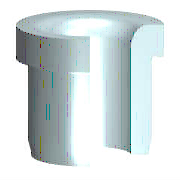
# Autodesk Inventor part: DIN 172 - A 3 x 12
Saved by Autodesk Inventor 2023.3 (Build 273359000, 359)
## iProperties
Created: 2022-02-04
Part Number: DIN 172 - A 3 x 12
Material: Stahl, weich
Description: Bohrbuchse
Document SubType Name: Modeling
Standard: DIN 172
Designer: nicob
Standards Organization: DIN
Language: de-DE
Size Designation: A 3 x 12
Categories: <MemberInstance><Categories><Category DisplayName="Sonstige Bauteile" InternalName="5aa15e00-363f-49f2-933f-16f664388e3f" Mnemonic="OTHER"><Category DisplayName="Bohrbuchsen" InternalName="dee9b2ed-98ff-44bf-b329-c7a8019090da" Mnemonic="BUSH"><CategoryParameter DisplayName="Max. Nenndurchmesser" InternalName="b1ee04ef-1694-415b-b3bc-4245da0f3d9b" Mnemonic="nomdiamax"/><CategoryParameter DisplayName="Nenndurchmesser" InternalName="b4c3aa1f-6c9b-46e9-b968-1f353908ad3b" Mnemonic="nomdia2"/><CategoryParameter DisplayName="Nennlänge" InternalName="c18b8459-7ef0-405c-9d91-ab742f171900" Mnemonic="nomlen2"/></Category></Category><Category DisplayName="Datentyp" InternalName="23b78d0f-2648-40c6-8793-ca6db495c9e8" Mnemonic="DATATYPE"><CategoryParameter DisplayName="Anzeigename" InternalName="05415f3d-3907-474b-a020-eb9d644f4cf3" Mnemonic="DISPLAYNAME"/><CategoryParameter DisplayName="Norm" InternalName="0c0a119c-1e12-4c84-803f-101930972f5e" Mnemonic="STANDARD"/><CategoryParameter DisplayName="Beschreibung" InternalName="13903e3d-64b1-4950-80da-f627842ea37f" Mnemonic="DESCRIPTION"/><CategoryParameter DisplayName="Bezeichnung" InternalName="2675968c-4ce5-49e0-a4f5-552d29089031" Mnemonic="DESIGNATION"/><CategoryParameter DisplayName="Standardzeile" InternalName="2af9ec52-faaa-4026-b378-f9fa4afca842" Mnemonic="DEFAULTROW"/><CategoryParameter DisplayName="Ordnername" InternalName="3f06958e-8713-4116-9be7-ed6184ecc97b" Mnemonic="FOLDERNAME"/><CategoryParameter DisplayName="Revisionsanleitung" InternalName="45a75005-10b1-4dfc-8d6d-dfe629f0b93c" Mnemonic="REVISIONGUID"/><CategoryParameter DisplayName="Dateiname" InternalName="8b46a4cc-9585-4fed-90c3-899f57e09a73" Mnemonic="FILENAME"/><CategoryParameter DisplayName="Normungsorganisation" InternalName="8f5914e1-4693-403f-8ab5-d37768198c9d" Mnemonic="STDSORG"/><CategoryParameter DisplayName="Gruppenversion" InternalName="914462f6-6e19-4b14-ba84-155b9680b1d0" Mnemonic="FAMILYREVISION"/><CategoryParameter DisplayName="Normrevision" InternalName="91d5a463-65c2-4fde-b823-3b7fea5e8e17" Mnemonic="STANDARDREVISION"/><CategoryParameter DisplayName="Variantenrevision" InternalName="a65d44b9-392f-4f4f-857b-e4b3d54996fe" Mnemonic="MEMBERREVISION"/><CategoryParameter DisplayName="ClipFormat" InternalName="bc51e27b-3422-4e78-93ef-cec197ddf230" Mnemonic="CLIPFORMAT"/><CategoryParameter DisplayName="Hersteller" InternalName="cd6c7a72-a28a-4e50-99a9-2c7f4e13e5ad" Mnemonic="MANUFACTURER"/><CategoryParameter DisplayName="InternerName" InternalName="cf1d0246-76d9-4b4a-8305-fa0409afb5c1" Mnemonic="INTERNALNAME"/><CategoryParameter DisplayName="IstMetrisch" InternalName="e2385c5b-1ea4-4823-96a8-8de651266ec3" Mnemonic="ISMETRIC"/><Category DisplayName="Bauteil" InternalName="c0e0b642-3bcb-4cc8-9e80-f96d35c4afa4" Mnemonic="PART"><CategoryParameter DisplayName="Bauteilnummer" InternalName="016b6077-bfbe-49bd-92c9-d8d59c39c941" Mnemonic="PARTNUMBER"/><CategoryParameter DisplayName="Bestandsnummer" InternalName="4dba7c1c-e26c-444e-836c-b08b433409a8" Mnemonic="STOCKNUMBER"/><CategoryParameter DisplayName="Materialschlüssel" InternalName="5c9a8adb-dd2b-4535-b97f-0a94a95fe41f" Mnemonic="MATERIALKEY"/><CategoryParameter DisplayName="Material" InternalName="818a152a-d3c3-49ca-80ee-df7d91421b8e" Mnemonic="MATERIAL"/></Category></Category><Category DisplayName="ÄltereVersionenzuweisen" InternalName="cd87c42b-3e48-431e-b5c0-1cbeb14dfe77" Mnemonic="LEGACYMAP"><CategoryParameter DisplayName="Eindeutige DA-Varianten-ID" InternalName="0918ad47-427f-4fed-ae26-24c81c58f590" Mnemonic="DACOOKIE"/><CategoryParameter DisplayName="ID zusammenführen" InternalName="0ee8fb18-e2ed-4f39-96f6-1f4b5f50aa71" Mnemonic="MERGE11"/><CategoryParameter DisplayName="Eindeutige CC-Varianten-ID" InternalName="5193edd4-b2b0-4ab4-9d54-de900eee34e0" Mnemonic="CCCOOKIE"/><CategoryParameter DisplayName="ID aufteilen" InternalName="72b5c83c-be7f-45c4-ae51-9160ea6deb26" Mnemonic="SPLIT"/><CategoryParameter DisplayName="VarianteID" InternalName="8e5e0294-fc51-4c8f-b3d7-003dc5ed94f6" Mnemonic="MEMBERID"/><CategoryParameter DisplayName="Katalogname" InternalName="d99d1e27-aa94-4de2-af4c-c348882a6f4f" Mnemonic="CATALOGNAME"/><CategoryParameter DisplayName="Gruppennummer" InternalName="e705e1f4-09cb-413e-91f9-551b4188271e" Mnemonic="FAMILYNUMBER"/></Category></Categories><FamilyTemplate Id="si0063"><FamilyTemplateParameters><FamilyTemplateParameter ObjectType="kUserParameterObject" ValueType="xs:double" Id="1" ObjectReferenceKey="KOH"/><FamilyTemplateParameter ObjectType="kUserParameterObject" ValueType="xs:double" Id="2" ObjectReferenceKey="NLG"/><FamilyTemplateParameter ObjectType="kUserParameterObject" ValueType="xs:double" Id="3" ObjectReferenceKey="KOD"/><FamilyTemplateParameter ObjectType="kUserParameterObject" ValueType="xs:double" Id="4" ObjectReferenceKey="PHH"/><FamilyTemplateParameter ObjectType="kUserParameterObject" ValueType="xs:double" Id="5" ObjectReferenceKey="NNDMIN"/><FamilyTemplateParameter ObjectType="kUserParameterObject" ValueType="xs:double" Id="6" ObjectReferenceKey="FSRR"/><FamilyTemplateParameter ObjectType="kUserParameterObject" ValueType="xs:double" Id="7" ObjectReferenceKey="RR"/><FamilyTemplateParameter ObjectType="kUserParameterObject" ValueType="xs:double" Id="8" ObjectReferenceKey="FST2"/><FamilyTemplateParameter ObjectType="kUserParameterObject" ValueType="xs:double" Id="9" ObjectReferenceKey="FST1"/><FamilyTemplateParameter ObjectType="kUserParameterObject" ValueType="xs:double" Id="10" ObjectReferenceKey="FSH"/><FamilyTemplateParameter ObjectType="kUserParameterObject" ValueType="xs:double" Id="11" ObjectReferenceKey="ANG"/><FamilyTemplateParameter ObjectType="kUserParameterObject" ValueType="xs:double" Id="12" ObjectReferenceKey="FSB"/><FamilyTemplateParameter ObjectType="kUserParameterObject" ValueType="xs:double" Id="13" ObjectReferenceKey="NNDMAX"/><FamilyTemplateParameter ObjectType="kUserParameterObject" ValueType="xs:double" Id="14" ObjectReferenceKey="NND"/><FamilyTemplateParameter ObjectType="kUserParameterObject" ValueType="xs:double" Id="15" ObjectReferenceKey="SEWI"/><FamilyTemplateParameter ObjectType="kUserParameterObject" ValueType="xs:double" Id="16" ObjectReferenceKey="SD2"/><FamilyTemplateParameter ObjectType="kPropertyObject" ValueType="xs:string" Id="100" ObjectReferenceKey="{32853F0F-3444-11d1-9E93-0060B03C1CA6}" SubObjectId="52"/><FamilyTemplateParameter ObjectType="kPropertyObject" ValueType="xs:string" Id="105" ObjectReferenceKey="{32853F0F-3444-11d1-9E93-0060B03C1CA6}" SubObjectId="5"/><FamilyTemplateParameter ObjectType="kPartComponentDefinitionObject" ValueType="xs:string" Id="110" SubObjectId="Material"/></FamilyTemplateParameters></FamilyTemplate><CategoryParameterMap><ParamToTemplateMap><ParamToTemplate CategoryParameter="//CategoryParameter[@InternalName='05415f3d-3907-474b-a020-eb9d644f4cf3']" ConstantValue="DIN 172 A"/><ParamToTemplate CategoryParameter="//CategoryParameter[@InternalName='cf1d0246-76d9-4b4a-8305-fa0409afb5c1']" ConstantValue="6643bd9c-a700-405d-9da7-12c75d06d1ae"/><ParamToTemplate CategoryParameter="//CategoryParameter[@InternalName='3f06958e-8713-4116-9be7-ed6184ecc97b']" ConstantValue="DIN 172  A"/><ParamToTemplate CategoryParameter="//CategoryParameter[@InternalName='914462f6-6e19-4b14-ba84-155b9680b1d0']" ConstantValue="10"/><ParamToTemplate CategoryParameter="//CategoryParameter[@InternalName='bc51e27b-3422-4e78-93ef-cec197ddf230']" ConstantValue="CF_INVENTOR.STDPARTS"/><ParamToTemplate CategoryParameter="//CategoryParameter[@InternalName='e2385c5b-1ea4-4823-96a8-8de651266ec3']" ConstantValue="true"/><ParamToTemplate CategoryParameter="//CategoryParameter[@InternalName='13903e3d-64b1-4950-80da-f627842ea37f']" ConstantValue="Press Fit Bushing"/><ParamToTemplate CategoryParameter="//CategoryParameter[@InternalName='8f5914e1-4693-403f-8ab5-d37768198c9d']" ConstantValue="DIN"/><ParamToTemplate CategoryParameter="//CategoryParameter[@InternalName='0c0a119c-1e12-4c84-803f-101930972f5e']" ConstantValue="DIN 172"/><ParamToTemplate CategoryParameter="//CategoryParameter[@InternalName='cd6c7a72-a28a-4e50-99a9-2c7f4e13e5ad']" TemplateParameter="104"/><ParamToTemplate CategoryParameter="//CategoryParameter[@InternalName='91d5a463-65c2-4fde-b823-3b7fea5e8e17']" TemplateParameter="103"/><ParamToTemplate CategoryParameter="//CategoryParameter[@InternalName='45a75005-10b1-4dfc-8d6d-dfe629f0b93c']" ConstantValue="72bfe220-aaac-4541-a17e-c3dc227c6a26"/><ParamToTemplate CategoryParameter="//CategoryParameter[@InternalName='2af9ec52-faaa-4026-b378-f9fa4afca842']" ConstantValue="10"/><ParamToTemplate CategoryParameter="//CategoryParameter[@InternalName='d99d1e27-aa94-4de2-af4c-c348882a6f4f']" ConstantValue="DIN"/><ParamToTemplate CategoryParameter="//CategoryParameter[@InternalName='e705e1f4-09cb-413e-91f9-551b4188271e']" ConstantValue="229"/><ParamToTemplate CategoryParameter="//CategoryParameter[@InternalName='8b46a4cc-9585-4fed-90c3-899f57e09a73']" ConstantValue="DIN 172 - A 3 x 12"/><ParamToTemplate CategoryParameter="//CategoryParameter[@InternalName='a65d44b9-392f-4f4f-857b-e4b3d54996fe']" ConstantValue="1F974138-520D-4115-B96C-7A635634038E"/><ParamToTemplate CategoryParameter="//CategoryParameter[@InternalName='8e5e0294-fc51-4c8f-b3d7-003dc5ed94f6']" ConstantValue="80"/><ParamToTemplate CategoryParameter="//CategoryParameter[@InternalName='2675968c-4ce5-49e0-a4f5-552d29089031']" TemplateParameter="100"/><ParamToTemplate CategoryParameter="//CategoryParameter[@InternalName='818a152a-d3c3-49ca-80ee-df7d91421b8e']" TemplateParameter="110"/><ParamToTemplate CategoryParameter="//CategoryParameter[@InternalName='c18b8459-7ef0-405c-9d91-ab742f171900']" TemplateParameter="2"/><ParamToTemplate CategoryParameter="//CategoryParameter[@InternalName='b4c3aa1f-6c9b-46e9-b968-1f353908ad3b']" TemplateParameter="14"/><ParamToTemplate CategoryParameter="//CategoryParameter[@InternalName='b1ee04ef-1694-415b-b3bc-4245da0f3d9b']" TemplateParameter="13"/><ParamToTemplate CategoryParameter="//CategoryParameter[@InternalName='016b6077-bfbe-49bd-92c9-d8d59c39c941']" TemplateParameter="105"/></ParamToTemplateMap></CategoryParameterMap></MemberInstance>
Mass: 2.5968 g
Surface Area: 4.72358 cm^2
Volume: 0.330803 cm^3
Density: 7.85 g/cm^3
Appearance: Halbpoliert
IsCustomPart: 1
Author: nicob
Autodesk Inventor part; units mm, degrees
ref_plane "YZ Plane" through (0, 0, 0) normal (1, 0, 0) x (0, 1, 0)
ref_plane "XZ Plane" through (0, 0, 0) normal (0, 1, 0) x (-1, 0, 0)
sketch "Skizze1" plane through (0, 0, 0) normal (0, 0, 1) x (1, 0, 0)
  line L0 (-2.5, 0) -> (5.5, 0)
  line L1 (9.5, 1.5) -> (9.5, 3)
  line L2 (9.5, 3) -> (2, 3)
  line L3 (-2.5, 1.5) -> (-2.5, 4.5)
  line L4 (-2.5, 4.5) -> (0, 4.5)
  line L5 (2, 3) -> (1.3045, 2.8136)
  line L6 (1.2009, 2.8) -> (0.3, 2.8)
  line L7 (-0.0913, 3.2832) -> (0, 3.7125)
  line L8 (0, 3.7125) -> (0, 4.5)
  arc A0 (-0.0913, 3.2832) -> (0.3, 2.8) centre (0.3, 3.2) ccw
  arc A1 (1.2009, 2.8) -> (1.3045, 2.8136) centre (1.2009, 3.2) ccw
  line L9 (-28.4, 0) -> (128.4, 0) projected
  line L10 (0, -12) -> (0, 72) projected
  line L11 (-2.5, 1.5) -> (9.5, 1.5)
  dimension "d0" = 9
  dimension "d1" = 6
  dimension "d2" = 12
  dimension "d3" = 12
  dimension "d4" = 0.4
  dimension "d5" = 0.1
  dimension "d6" = 2
  dimension "d7" = 15
  dimension "d8" = 0.2
  dimension "d9" = 0.4
  dimension "d10" = 2.5
  dimension "d11" = 3
  constraints: 20 end point, 5 perpendicular, 4 point on circle, 4 tangent, 2 centre point, 2 collinear, 2 horizontal, 2 parallel
  measures "d0" diameter of L4 L0
  measures "d1" diameter of L2 L0
  measures "d2" distance between parallel lines of L1 L3
  measures "d3" angle of L8 L7
  measures "d4" radius of A0
  measures "d5" distance edge to line of A0 L8
  measures "d6" distance from line of L2.end L8
  measures "d7" angle of L2 L5
  measures "d8" distance between parallel lines of L6 L2
  measures "d9" radius of A1
  measures "d10" distance between parallel lines of L8 L3
  measures "d11" diameter of L11 L0
revolve "Körper" add sketch "Skizze1" angle 360 about axis through (-2.5, 0, 0) along (1, 0, 0) contours L11 L10 A0 L6 A1 L5 L2 L1 | L11 L3 L4 L8 L7 A0 L10
chamfer "Fase1" distance 1 angle 15 1 edges at (9.5, -3, 0) measured on face at (9, -3, 0)
fillet "Rundung1" radius 1 1 edges at (-2.5, -1.5, 0)
ref_plane "Arbeitsebene1" through (0, 0, 3) normal (0, 0, 1) x (1, 0, 0)
sketch "Skizze2" plane through (0, 0, 3) normal (0, 0, 1) x (1, 0, 0)
  line L0 (9.5, 2.7321) -> (9.5, -2.7321) projected
  line L1 (-2.5, -4.5) -> (-2.5, 4.5) projected
  point P0 (0, 0)
  point P1 (3.5, 0)
  point P2 (9.5, 0)
  dimension "d39" = 6
  constraints: 1 horizontal alignment, 1 midpoint
  measures "d39" distance from line of point (3.5, 0) L1
hole "Bohrung1" at (3.5, 0, 3) direction (0, 0, -1) diameter 0.5 end through all
equation "\"d12\" = PHH"
equation "\"d13\" = ANG"
equation "\"d29\" = PHH"
equation "\"d14\" = RR"
equation "\"d0\" = KOD"
equation "\"d1\" = SD2"
equation "\"d2\" = NLG"
equation "\"d4\" = FSRR"
equation "\"d5\" = FST2"
equation "\"d6\" = FSB"
equation "\"d8\" = FST1"
equation "\"d9\" = FSRR"
equation "\"d10\" = KOH"
equation "\"d11\" = NND"
equation "\"NLG\" = 12"
equation "\"NND\" = 3"
equation "\"KOD\" = 9"
equation "\"KOH\" = 2.5"
equation "\"SD2\" = 6"
equation "\"FST1\" = 0.2"
equation "\"FST2\" = 0.1"
equation "\"FSB\" = 2"
equation "\"FSRR\" = 0.4"
equation "\"PHH\" = 1"
equation "\"ANG\" = 15deg"
equation "\"RR\" = 1"
equation "\"NNDMIN\" = 2.7"
equation "\"FSH\" = 1.1"
equation "\"NNDMAX\" = 3.3"
equation "\"SEWI\" = 30deg"
body "Solid1"
